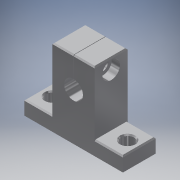
# Autodesk Inventor part: SK12
Saved by Autodesk Inventor 2017 (Build 210142000, 142)
## iProperties
Part Number: SK12
Material: Aluminium 5005
Document SubType Name: Modeling
Designer: Till
Density: 2.7 g/cm^3
Appearance: Aluminium - dunkel
Author: Till
Autodesk Inventor part; units mm, degrees
ref_plane "YZ Plane" through (0, 0, 0) normal (1, 0, 0) x (0, 1, 0)
ref_plane "XZ Plane" through (0, 0, 0) normal (0, 1, 0) x (-1, 0, 0)
ref_plane "XY Plane" through (0, 0, 0) normal (0, 0, 1) x (1, 0, 0)
sketch "Skizze1" plane through (0, 0, 0) normal (0, 0, 1) x (1, 0, 0)
  line L0 (21, 7) -> (-21, 7)
  line L1 (-21, 7) -> (-21, -7)
  line L2 (-21, -7) -> (21, -7)
  line L3 (21, -7) -> (21, 7)
  line L4 (21, 7) -> (-21, -7) construction
  line L5 (-21, 7) -> (21, -7) construction
  point P0 (0, 0)
  dimension "d0" = 42
  dimension "d1" = 14
  constraints: 12 end point, 2 midpoint, 2 parallel, 1 horizontal, 1 perpendicular
  measures "d0" distance of L2.end L1.end
  measures "d1" distance of L1.end L0.end
extrude "Extrusion1" add sketch "Skizze1" along normal blind 6
sketch "Skizze2" plane through (0, 0, 6) normal (0, 0, 1) x (1, 0, 0)
  line L0 (21, 7) -> (-21, 7) projected
  line L1 (-9, -7) -> (9, -7)
  line L2 (9, -7) -> (9, 7)
  line L3 (9, 7) -> (-9, 7)
  line L4 (-9, 7) -> (-9, -7)
  line L5 (-9, -7) -> (9, 7) construction
  line L6 (9, -7) -> (-9, 7) construction
  point P0 (0, 0)
  dimension "d4" = 18
  constraints: 12 end point, 2 midpoint, 2 parallel, 1 horizontal, 1 perpendicular, 1 point on line
  measures "d4" distance of L3.end L2.end
extrude "Extrusion2" add sketch "Skizze2" along normal blind 26.8
sketch "Skizze3" plane through (-21, -7, 0) normal (0, -1, 0) x (1, 0, 0)
  line L0 (20.8889, 32.8) -> (20.8889, 23.9985)
  line L1 (21.1111, 32.8) -> (21.1111, 23.9985)
  arc A0 (20.8889, 23.9985) -> (21.1111, 23.9985) centre (21, 20) ccw
  line L2 (20.8889, 32.8) -> (21.1111, 32.8)
  line L3 (0, 0) -> (42, 0) projected
  line L4 (12, 32.8) -> (30, 32.8) projected
  point P0 (21, 0)
  dimension "d28" = 20
  dimension "d29" = 4
  dimension "d30" = 0
  constraints: 6 end point, 2 point on circle, 1 centre point, 1 parallel
  measures "d28" distance from line of L3 A0.centre
  measures "d29" radius of A0
  measures "d30" distance between parallel lines of L2 L4
extrude "Extrusion3" cut sketch "Skizze3" against normal through all
sketch "Skizze4" plane through (9, -7, 6) normal (1, 0, 0) x (0, 0, -1)
  circle A0 centre (-22.3, 7) radius 2.25
  line L0 (-26.8, 0) -> (-26.8, 14) projected
  point P0 (6, 7)
  dimension "d13" = 4.5
  dimension "d31" = 4.5
  constraints: 1 centre point
  measures "d13" diameter of A0
  measures "d31" distance from line of L0 A0.centre
extrude "Extrusion4" cut sketch "Skizze4" against normal through all
sketch "Skizze5" plane through (9, -7, 6) normal (1, 0, 0) x (0, 0, -1)
  circle A0 centre (-22.3, 7) radius 2.25 projected
  circle A1 centre (-22.3, 7) radius 3.75
  point P0 (6, 7)
  dimension "d16" = 7.5
  constraints: 1 centre point, 1 coincident
  measures "d16" diameter of A1
extrude "Extrusion5" cut sketch "Skizze5" against normal blind 3.5
sketch "Skizze6" plane through (0, 0, 6) normal (0, 0, 1) x (1, 0, 0)
  circle A0 centre (16, 0) radius 2.75
  circle A1 centre (-16, 0) radius 2.75
  line L0 (-21, 7) -> (-21, -7) projected
  point P0 (0, 0)
  dimension "d19" = 5.5
  dimension "d20" = 5.5
  dimension "d21" = 32
  dimension "d22" = 5
  constraints: 2 centre point
  measures "d19" diameter of A0
  measures "d20" diameter of A1
  measures "d21" distance of A0.centre A1.centre
  measures "d22" distance from line of L0 A1.centre
extrude "Extrusion6" cut sketch "Skizze6" against normal up to next
chamfer "Fase1" distance 0.5 angle 45 14 edges at (21, 0, 6) (-21, 0, 6) (15, 7, 6) (-15, 7, 6) (-15, -7, 6) (15, -7, 6) (9, 0, 32.8) (-9, 0, 32.8) (-4.5556, -7, 32.8) (4.5556, -7, 32.8) (4.5556, 7, 32.8) (-4.5556, 7, 32.8) (13.25, 0, 6) (-18.75, 0, 6)
